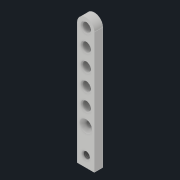
# Autodesk Inventor part: Pivot Leg
Saved by Autodesk Inventor 2021.1 (Build 251245000, 245)
## iProperties
Created: 2020-05-07
Part Number: Pivot Leg
Material: Generic
Document SubType Name: Modeling
Designer: Workshop Tech
Density: 1 g/cm^3
Appearance: Default
Author: Workshop Tech
Autodesk Inventor part; units mm, degrees
ref_plane "YZ Plane" through (0, 0, 0) normal (1, 0, 0) x (0, 1, 0)
ref_plane "XZ Plane" through (0, 0, 0) normal (0, 1, 0) x (-1, 0, 0)
ref_plane "XY Plane" through (0, 0, 0) normal (0, 0, 1) x (1, 0, 0)
sketch "Sketch1" plane through (0, 0, 0) normal (0, 0, 1) x (1, 0, 0)
  line L0 (0, 0) -> (12.7, 0)
  line L1 (12.7, 0) -> (12.7, 96.8375)
  line L2 (12.7, 96.8375) -> (0, 96.8375)
  line L3 (0, 96.8375) -> (0, 0)
  dimension "d0" = 12.7
  dimension "d1" = 96.8375
  constraints: 8 end point, 2 parallel, 1 horizontal, 1 perpendicular
  measures "d0" distance between parallel lines of L1 L3
  measures "d1" distance between parallel lines of L0 L2
extrude "Body" add sketch "Sketch1" along normal blind 6.35
sketch "Sketch2" plane through (0, 0, 6.35) normal (0, 0, 1) x (1, 0, 0)
  line L0 (12.7, 0) -> (12.7, 96.8375) projected
  line L1 (0, 0) -> (12.7, 0) projected
  point P0 (6.35, 7.62)
  dimension "d4" = 6.35
  dimension "d5" = 7.62
  measures "d4" distance from line of L0 point (6.35, 7.62)
  measures "d5" distance from line of L1 point (6.35, 7.62)
hole "QBot Mount Hole" at (6.35, 7.62, 6.35) direction (0, 0, -1) diameter 4.9276 end through all countersink diameter 6.35 countersink angle 90
sketch "Sketch3" plane through (0, 0, 6.35) normal (0, 0, 1) x (1, 0, 0)
  line L0 (12.7, 0) -> (12.7, 96.8375) projected
  circle A0 centre (6.35, 7.62) radius 3.2004
  line L1 (0, 0) -> (12.7, 0) projected
  point P0 (6.35, 26.67)
  dimension "d13" = 6.35
  dimension "d14" = 19.05
  dimension "d35" = 6.4008
  dimension "d36" = 7.62
  constraints: 1 centre point, 1 vertical alignment
  measures "d13" distance from line of L0 point (6.35, 26.67)
  measures "d14" distance of point (6.35, 26.67) A0.centre
  measures "d35" diameter of A0
  measures "d36" distance from line of L1 A0.centre
hole "Plate Mount Hole" at (6.35, 26.67, 6.35) direction (0, 0, -1) diameter 4.2926 end through all countersink diameter 9.398 countersink angle 90 clearance for "Countersunk Flat Head Screw ISO 2009/7046" size "M4" standard "ISO"
sketch "Sketch4" plane through (0, 0, 6.35) normal (0, 0, 1) x (1, 0, 0)
  line L0 (12.7, 0) -> (12.7, 96.8375) projected
  circle A0 centre (6.35, 26.67) radius 2.1463 projected
  point P0 (0, 0)
  point P1 (6.35, 39.37)
  dimension "d22" = 6.35
  dimension "d23" = 12.7
  measures "d22" distance from line of L0 point (6.35, 39.37)
  measures "d23" distance of point (6.35, 39.37) A0.centre
hole "Axle Hole" at (6.35, 39.37, 6.35) direction (0, 0, -1) diameter 6.35 end through all
pattern_linear "Rectangular Pattern1" count 5 spacing 12.7 along (0, 1, 0) of "Axle Hole"
fillet "Fillet1" radius 6.35 2 edges at (12.7, 96.8375, 3.175) (0, 96.8375, 3.175)
chamfer "Chamfer1" distance 0.7937 angle 45 5 edges at (6.35, 42.545, 6.35) (6.35, 55.245, 6.35) (6.35, 67.945, 6.35) (6.35, 80.645, 6.35) (6.35, 93.345, 6.35)
body "Solid1"
